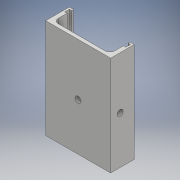
# Autodesk Inventor part: Pcam5C_holder
Saved by Autodesk Inventor 2018 (Build 220112000, 112)
## iProperties
Created: 2018-04-27
Part Number: Pcam5C_holder
Material: 一般
Document SubType Name: Modeling
Designer: izumi
Density: 1 g/cm^3
Appearance: 既定
Author: izumi
Autodesk Inventor part; units mm, degrees
ref_plane "YZ Plane" through (0, 0, 0) normal (1, 0, 0) x (0, 1, 0)
ref_plane "XZ Plane" through (0, 0, 0) normal (0, 1, 0) x (-1, 0, 0)
ref_plane "XY Plane" through (0, 0, 0) normal (0, 0, 1) x (1, 0, 0)
sketch "本体面" plane through (0, 0, 0) normal (0, 0, 1) x (1, 0, 0)
  line L0 (-13.7, 10) -> (13.7, 10)
  line L1 (13.7, 10) -> (13.7, 0)
  line L2 (13.7, 0) -> (-13.7, 0)
  line L3 (-13.7, 0) -> (-13.7, 10)
  point P0 (0, 0)
  point P1 (0, 0)
  dimension "d0" = 27.4
  dimension "d1" = 10
  constraints: 8 end point, 2 parallel, 1 coincident, 1 horizontal, 1 midpoint, 1 perpendicular
  measures "d0" distance of L1.end L2.end
  measures "d1" distance of L0.end L1.end
extrude "本体" add sketch "本体面" along normal blind 42
sketch "空洞面" plane through (0, 0, 42) normal (0, 0, 1) x (1, 0, 0)
  line L0 (-11.9, 10) -> (11.9, 10)
  line L1 (11.9, 10) -> (11.9, 3.5)
  line L2 (9.9, 1.5) -> (-9.9, 1.5)
  line L3 (-11.9, 3.5) -> (-11.9, 10)
  line L4 (13.7, 10) -> (-13.7, 10) projected
  arc A0 (-11.9, 3.5) -> (-9.9, 1.5) centre (-9.9, 3.5) ccw
  arc A1 (9.9, 1.5) -> (11.9, 3.5) centre (9.9, 3.5) ccw
  point P0 (0, 0)
  point P1 (11.9, 1.5)
  point P2 (-11.9, 1.5)
  point P3 (0, 10)
  dimension "d4" = 23.8
  dimension "d5" = 8.5
  dimension "d6" = 2
  constraints: 8 end point, 4 point on circle, 4 point on line, 4 tangent, 2 centre point, 2 midpoint, 2 parallel, 1 equal radius, 1 horizontal, 1 perpendicular
  measures "d4" distance of point (11.9, 1.5) point (-11.9, 1.5)
  measures "d5" distance of L0.end point (11.9, 1.5)
  measures "d6" radius of A0
extrude "空洞" cut sketch "空洞面" against normal blind 42
sketch "左溝面" plane through (0, 0, 42) normal (0, 0, 1) x (1, 0, 0)
  line L0 (-12.9, 9.2) -> (-11.9, 9.2)
  line L1 (-11.9, 9.2) -> (-11.9, 7.2)
  line L2 (-11.9, 7.2) -> (-12.9, 7.2)
  line L3 (-12.9, 7.2) -> (-12.9, 9.2)
  line L4 (-11.9, 10) -> (-13.7, 10) construction
  line L5 (-13.7, 10) -> (-13.7, 0) construction
  line L6 (-11.9, 3.5) -> (-11.9, 10) construction
  point P0 (0, 0)
  dimension "d10" = 2
  dimension "d27" = 0.8
  dimension "d28" = 0.8
  constraints: 8 end point, 2 parallel, 1 collinear, 1 horizontal, 1 perpendicular
  measures "d10" distance of L0.end L1.end
  measures "d27" distance between parallel lines of L0 L4
  measures "d28" distance between parallel lines of L3 L5
extrude "左溝" cut sketch "左溝面" against normal blind 41
sketch "右溝面" plane through (0, 0, 42) normal (0, 0, 1) x (1, 0, 0)
  line L0 (11.9, 9.2) -> (12.9, 9.2)
  line L1 (12.9, 9.2) -> (12.9, 7.2)
  line L2 (12.9, 7.2) -> (11.9, 7.2)
  line L3 (11.9, 7.2) -> (11.9, 9.2)
  line L4 (13.7, 10) -> (11.9, 10) projected
  line L5 (13.7, 0) -> (13.7, 10) projected
  line L6 (11.9, 10) -> (11.9, 3.5) projected
  point P0 (0, 0)
  dimension "d22" = 2
  dimension "d29" = 0.8
  dimension "d30" = 0.8
  constraints: 8 end point, 2 parallel, 1 collinear, 1 horizontal, 1 perpendicular
  measures "d22" distance of L2.end L0.start
  measures "d29" distance between parallel lines of L4 L0
  measures "d30" distance between parallel lines of L5 L1
extrude "右溝" cut sketch "右溝面" against normal blind 41
sketch "右穴位置" plane through (13.7, 0, 0) normal (1, 0, 0) x (0, 0, -1)
  line L0 (-20, 0) -> (0, 0) construction
  line L1 (-20, 0) -> (-20, 4) construction
  line L2 (0, 10) -> (-42, 10) construction
  line L3 (0, 0) -> (-42, 0) construction
  line L4 (0, 10) -> (0, 0) construction
  dimension "d31" = 20
  dimension "d32" = 4
  constraints: 4 end point, 1 coincident, 1 horizontal, 1 vertical
  measures "d31" distance of L0.end L0.start
  measures "d32" distance of L0.start L1.end
hole "右穴" at (13.7, 4, 20) direction (-1, 0, 0) diameter 2.5 depth 8 tip angle 118
sketch "左穴位置" plane through (-13.7, 0, 0) normal (-1, 0, 0) x (0, 0, 1)
  line L0 (0, 0) -> (20, 0) construction
  line L1 (20, 0) -> (20, 4) construction
  point P0 (0, 0)
  point P1 (0, 0)
  dimension "d40" = 4
  dimension "d41" = 20
  constraints: 4 coincident, 4 end point, 1 horizontal, 1 vertical
  measures "d40" distance of L0.end L1.end
  measures "d41" distance of L0.start L0.end
hole "左穴" at (-13.7, 4, 20) direction (1, 0, 0) diameter 2.5 depth 8 tip angle 118
sketch "背穴位置" plane through (-13.7, 0, 0) normal (0, -1, 0) x (1, 0, 0)
  line L0 (13.7, 20) -> (13.7, 0) construction
  line L1 (27.4, 0) -> (0, 0) construction
  dimension "d49" = 20
  constraints: 2 end point, 1 coincident, 1 midpoint, 1 vertical
  measures "d49" distance of L0.start L0.end
hole "背穴" at (0, 0, 20) direction (0, 1, 0) diameter 2.5 depth 8 tip angle 118
